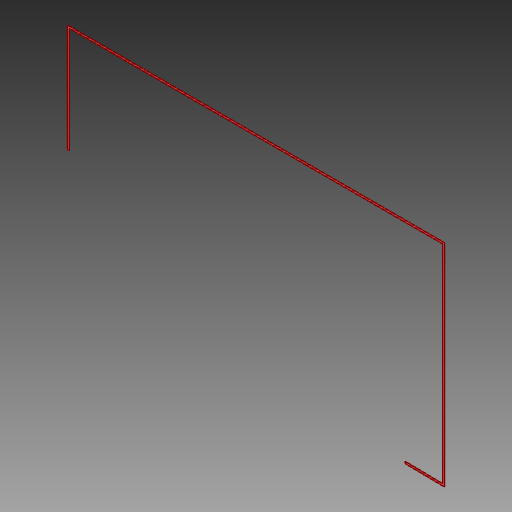
# Autodesk Inventor part: Trim-Red_03
Saved by Autodesk Inventor 2017.1 (Build 211199000, 199)
## iProperties
Created: 2017-01-08
Part Number: Trim-Red_03
Material: Generic
Document SubType Name: Modeling
Designer: PhillipD
Density: 1 g/cm^3
Appearance: Smooth - Red
Author: PhillipD
Autodesk Inventor part; units mm, degrees
ref_plane "YZ Plane" through (0, 0, 0) normal (1, 0, 0) x (0, 1, 0)
ref_plane "XZ Plane" through (0, 0, 0) normal (0, 1, 0) x (-1, 0, 0)
ref_plane "Work Plane1" through (0, 0, 0) normal (0, 0, 1) x (1, 0, 0)
sketch "Sketch1" plane through (0, 0, 0) normal (0, 0, 1) x (1, 0, 0)
  line L0 (-6858, 11887.2) -> (-2286, 11887.2) projected
  line L1 (-6858, -11887.2) -> (-6858, 11887.2) projected
  line L2 (2286, 11887.2) -> (2286, -11887.2) projected
  line L3 (-2286, 11887.2) -> (2286, 11887.2) projected
  line L4 (-6858, 11887.2) -> (2921, 11887.2)
  line L5 (2921, 11887.2) -> (2921, 6400.8)
  line L6 (-6858, 9091.6125) -> (2286, 9091.6125) projected
  line L7 (-6858, 11887.2) -> (-6858, 9091.6125)
  line L8 (1899.158, 4586.3002) -> (1899.158, 6415.1002) projected
  line L9 (2921, 6400.8) -> (1899.158, 6415.1002)
  line L10 (1899.8689, 6465.8952) -> (2870.2, 6452.3159)
  line L11 (2870.2, 6452.3159) -> (2870.2, 11836.4)
  line L12 (2870.2, 11836.4) -> (-6807.2, 11836.4)
  line L13 (-6807.2, 11836.4) -> (-6807.2, 9091.6125)
  line L14 (1899.158, 6415.1002) -> (1899.8689, 6465.8952)
  line L15 (-6858, 9091.6125) -> (-6807.2, 9091.6125)
  line L16 (1899.158, 6415.1002) -> (1899.8689, 6465.8952)
  point P0 (0, 0)
  dimension "d0" = 9779
  dimension "d1" = 5486.4
  dimension "d2" = 50.8
  constraints: 22 end point, 3 perpendicular, 2 collinear, 1 horizontal, 1 vertical, 2 other
  measures "d0" distance of L0.start L4.end
  measures "d1" distance of L4.end L5.end
  measures "d2" distance between parallel lines of L5 L11
extrude "Extrusion1" add sketch "Sketch1" along normal blind 6.35 contours L0 L3 L2 L12 L13 L6 L1 | L4 L5 L9 L2 L10 L11 L12 | L2 L9 L14 L10
body "Solid1"
